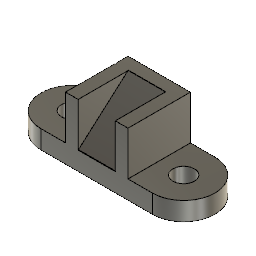
A2 v1 (Autodesk Fusion 360 design; units mm, degrees)
Autodesk Fusion 360 part; units mm, degrees
sketch "Sketch1" plane through (0, 0, 0) normal (0, 0, 1) x (1, 0, 0)
  line L0 (57, 32) -> (-57, 32)
  line L1 (-57, -32) -> (57, -32)
  circle A0 centre (57, 0) radius 11
  circle A1 centre (-57, 0) radius 11
  line L2 (-32, 32) -> (32, 32)
  line L3 (32, 32) -> (32, 19)
  line L4 (-32, 19) -> (-32, 32)
  arc A2 (-31.2512, 19) -> (-32, 19.975) centre (-57, 0) ccw
  arc A3 (-57, 32) -> (-57, -32) centre (-57, 0) ccw
  arc A4 (57, -32) -> (57, 32) centre (57, 0) ccw
  line L5 (-32, 19) -> (-31.2512, 19)
  line L6 (-19, 19) -> (-19, -32)
  line L7 (-19, -32) -> (-32, -32)
  line L8 (-32, -32) -> (-32, 19)
  line L9 (32, 19) -> (31.2512, 19)
  line L10 (19, 19) -> (19, -32)
  line L11 (19, -32) -> (32, -32)
  line L12 (32, -32) -> (32, 19)
  line L13 (-32, 17.9649) -> (-29.6806, 16.6628) construction
  line L14 (-31.2512, 19) -> (-32, 19)
  line L15 (32, 19) -> (31.2512, 19)
  line L16 (19, 19) -> (-19, 19)
  dimension "d1" = 114
  dimension "d2" = 64
  dimension "d3" = 22
  dimension "d4" = 22
  dimension "d5" = 64
  dimension "d6" = 13
  dimension "d8" = 13
  dimension "d9" = 13
  constraint horizontal L0
  constraint parallel L0 L1
  constraint coincident origin L13
  constraint coincident L0.end A2
  constraint concentric A0 A4
  constraint concentric A1 A2
  constraint horizontal L2
  constraint vertical L3
  constraint horizontal L15
  constraint vertical L4
  constraint coincident L0 L2.start
  constraint coincident L4 A2.end
  constraint concentric A2 A3
  constraint horizontal L5
  constraint vertical L6
  constraint horizontal L7
  constraint vertical L8
  constraint horizontal L9
  constraint vertical L10
  constraint horizontal L11
  constraint vertical L12
  constraint coincident L8 L13.start
  constraint collinear L14 L15
  constraint collinear L15 L16
  measures "d1" distance of L1.start L1.end
  measures "d2" distance of L0.end L1.start
  measures "d3" diameter of A0
  measures "d4" diameter of A1
  measures "d5" distance of L2.start L2.end
  measures "d6" distance of L2.start L4.start
  measures "d8" distance of L4.start L6.start
  measures "d9" distance of L3.end L10.start
extrude "Extrude1" add sketch "Sketch1" along normal blind 19 contours L0 L1 L3 A4 L12 makes body 1
extrude "Extrude2" add sketch "Sketch1" along normal blind 19 separate body contours L0 L1 L4 A3 L8 makes body 2
extrude "Extrude3" add sketch "Sketch1" along normal blind 19 separate body contours L1 L6 L10 L16 makes body 3
sketch "Sketch2" plane through (0, 0, 0) normal (1, 0, 0) x (0, 1, 0)
  line L0 (-31.7021, 19.3192) -> (19.2979, 19.3192)
  line L1 (19.2979, 19.3192) -> (19.2979, 64.3192)
  line L2 (19.2979, 64.3192) -> (-31.7021, 19.3192)
  dimension "d16" = 51
  dimension "d17" = 45
  constraint horizontal L0
  constraint perpendicular L0 L1
  measures "d16" distance of L0.start L0.end
  measures "d17" distance of L0.end L1.end
extrude "Extrude4" add sketch "Sketch1" along normal blind 64 contours L0 L1 L2 L3 L4 A2 L5 L6 L7 L8 L10 L11 L12 L14 L16 bodies 1 2 3
extrude "Extrude5" add sketch "Sketch2" along normal mid plane 38 bodies 1
equation "d6 = 64 mm - 51 mm"
equation "d17 = 64 mm - 19 mm"
named bodies: "A2"
